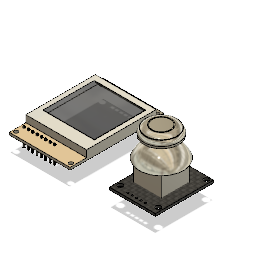
Paramotor_Instrument_Box-v4 (Autodesk Fusion 360 archive; units mm, degrees)
design "Burner Controller"
Autodesk Fusion 360 part; units mm, degrees
sketch "LCD_PCB" plane through (0, 0, 0) normal (0, 1, 0) x (1, 0, 0) in component "LCD Screen"
  line L0 (17.5, 27) -> (-17.5, 27)
  line L1 (-17.5, 27) -> (-17.5, -27)
  line L2 (-17.5, -27) -> (17.5, -27)
  line L3 (17.5, -27) -> (17.5, 27)
  line L4 (17.5, 27) -> (-17.5, -27) construction
  line L5 (-17.5, 27) -> (17.5, -27) construction
  circle A0 centre (-15.75, 24.75) radius 1.125
  circle A1 centre (15.75, 24.75) radius 1.125
  circle A2 centre (-15.75, -24.75) radius 1.125
  circle A3 centre (15.75, -24.75) radius 1.125
  circle A4 centre (0, 25) radius 0.5
  circle A5 centre (-10, 25) radius 0.5
  circle A6 centre (-7.5, 25) radius 0.5
  circle A7 centre (-5, 25) radius 0.5
  circle A8 centre (-2.5, 25) radius 0.5
  circle A9 centre (2.5, 25) radius 0.5
  circle A10 centre (5, 25) radius 0.5
  circle A11 centre (7.5, 25) radius 0.5
  circle A12 centre (10, 25) radius 0.5
  circle A13 centre (-15.5, -20) radius 0.5
  circle A14 centre (-13, -20) radius 0.5
  circle A15 centre (-10.5, -20) radius 0.5
  circle A16 centre (-8, -20) radius 0.5
  circle A17 centre (-5.5, -20) radius 0.5
  circle A18 centre (-3, -20) radius 0.5
  circle A19 centre (-0.5, -20) radius 0.5
  circle A20 centre (2, -20) radius 0.5
  dimension "d14" = 54
  dimension "d15" = 35
  dimension "d16" = 2.25
  dimension "d17" = 2.25
  dimension "d18" = 1.75
  dimension "d19" = 2.25
  dimension "d20" = 2.25
  dimension "d21" = 1.75
  dimension "d22" = 2.25
  dimension "d23" = 2.25
  dimension "d24" = 1.75
  dimension "d25" = 2.25
  dimension "d26" = 1.75
  dimension "d27" = 2.25
  dimension "d53" = 1
  dimension "d54" = 2
  dimension "d57" = 2.5
  dimension "d58" = 0
  dimension "d61" = 1
  dimension "d62" = 2
  dimension "d63" = 7
  dimension "d66" = 2.5
  dimension "d67" = 0
  constraint perpendicular L0 L1
  constraint parallel L0 L2
  constraint parallel L1 L3
  constraint horizontal L0
  constraint coincident L4 origin
  constraint coincident L5 origin
  measures "d14" distance of L0.end L1.end
  measures "d15" distance of L1.end L2.end
  measures "d16" diameter of A0
  measures "d17" distance of L0 A0.centre
  measures "d18" distance of L1 A0.centre
  measures "d19" diameter of A1
  measures "d20" distance of L0 A1.centre
  measures "d21" distance of L3 A1.centre
  measures "d22" diameter of A2
  measures "d23" distance of L2 A2.centre
  measures "d24" distance of L1 A2.centre
  measures "d25" diameter of A3
  measures "d26" distance of L3 A3.centre
  measures "d27" distance of L2 A3.centre
  measures "d53" diameter of A4
  measures "d54" distance of L0 A4.centre
  measures "d61" diameter of A13
  measures "d62" distance of L1 A13.centre
  measures "d63" distance of L2 A13.centre
extrude "Extrude1" add sketch "LCD_PCB" along normal blind 1.5 makes body 1 in component "LCD Screen"
sketch "LCD_Display" plane through (0, 1.5, 0) normal (0, 1, 0) x (-1, 0, 0) in component "LCD Screen"
  circle A0 centre (15.75, 24.75) radius 1.125
  circle A1 centre (-15.75, 24.75) radius 1.125
  circle A2 centre (-15.75, -24.75) radius 1.125
  circle A3 centre (15.75, -24.75) radius 1.125
  line L0 (-17.5, 27) -> (-17.5, -27)
  line L1 (-17.5, -27) -> (17.5, -27)
  line L2 (17.5, -27) -> (17.5, 27)
  line L3 (17.5, 27) -> (-17.5, 27)
  line L4 (-17.5, -22.5) -> (17.5, -22.5)
  line L5 (17.5, -22.5) -> (17.5, 17.5)
  line L6 (17.5, 17.5) -> (-17.5, 17.5)
  line L7 (-17.5, 17.5) -> (-17.5, -22.5)
  line L8 (-17.5, -22.5) -> (17.5, 17.5) construction
  line L9 (17.5, -22.5) -> (-17.5, 17.5) construction
  line L10 (14.75, -19.2) -> (-14.75, -19.2)
  line L11 (-14.75, -19.2) -> (-14.75, 10.3)
  line L12 (-14.75, 10.3) -> (14.75, 10.3)
  line L13 (14.75, 10.3) -> (14.75, -19.2)
  line L14 (14.75, -19.2) -> (-14.75, 10.3) construction
  line L15 (-14.75, -19.2) -> (14.75, 10.3) construction
  circle A4 centre (0, -25) radius 0.5
  circle A5 centre (-10, -25) radius 0.5
  circle A6 centre (-7.5, -25) radius 0.5
  circle A7 centre (-5, -25) radius 0.5
  circle A8 centre (-2.5, -25) radius 0.5
  circle A9 centre (2.5, -25) radius 0.5
  circle A10 centre (5, -25) radius 0.5
  circle A11 centre (7.5, -25) radius 0.5
  circle A12 centre (10, -25) radius 0.5
  circle A13 centre (-7.5, -25) radius 0.5
  circle A14 centre (-5, -25) radius 0.5
  circle A15 centre (-2.5, -25) radius 0.5
  circle A16 centre (-10, -25) radius 0.5
  circle A17 centre (2.5, -25) radius 0.5
  circle A18 centre (5, -25) radius 0.5
  circle A19 centre (7.5, -25) radius 0.5
  circle A20 centre (0, -25) radius 0.5
  circle A21 centre (10, -25) radius 0.5
  circle A22 centre (0.5, 20) radius 0.5
  circle A23 centre (-2, 20) radius 0.5
  circle A24 centre (13, 20) radius 0.5
  circle A25 centre (8, 20) radius 0.5
  circle A26 centre (5.5, 20) radius 0.5
  circle A27 centre (3, 20) radius 0.5
  circle A28 centre (10.5, 20) radius 0.5
  circle A29 centre (15.5, 20) radius 0.5
  point P0 (0, -2.5)
  point P1 (0, -4.45)
  dimension "d30" = 35
  dimension "d31" = 40
  dimension "d32" = 4.5
  dimension "d33" = 29.5
  dimension "d34" = 29.5
  dimension "d36" = 3.3
  dimension "d47" = 1
  dimension "d48" = 2
  dimension "d51" = 2.5
  dimension "d52" = 2.5
  constraint perpendicular L4 L5
  constraint parallel L4 L6
  constraint parallel L5 L7
  constraint horizontal L4
  constraint coincident L8 P0
  constraint coincident L9 P0
  constraint perpendicular L10 L11
  constraint parallel L10 L12
  constraint parallel L11 L13
  constraint horizontal L10
  constraint coincident L14 P1
  constraint coincident L15 P1
  measures "d30" distance of L5.end L6.end
  measures "d31" distance of L4.end L5.end
  measures "d32" distance of L1 L4
  measures "d33" distance of L11.end L12.end
  measures "d34" distance of L10.end L11.end
  measures "d36" distance of L4 L10
  measures "d47" diameter of A4
  measures "d48" distance of L1 A4.centre
extrude "Extrude2" add sketch "LCD_Display" along normal blind 4 contours L0 L2 L4 L5 L6 L7 bodies 1 in component "LCD Screen"
extrude "Extrude3" add 1 faces at (-4.9167, 1.5, -9.3667) along direction (0, 1, 0) blind 4.1 on bodies 1 bodies 1 in component "LCD Screen"
fillet "Fillet1" radius 0.1 4 edges at (0, 5.5, 10.3) (14.75, 5.5, -4.45) (0, 5.5, -19.2) (-14.75, 5.5, -4.45) on bodies 1 in component "LCD Screen"
sketch "Pins" plane through (0, 0, 0) normal (0, 1, 0) x (-1, 0, 0) in component "LCD Screen"
  line L0 (-16.5, 11.5) -> (-16.5, -21.5)
  line L1 (-16.5, -21.5) -> (16.5, -21.5)
  line L2 (16.5, -21.5) -> (16.5, 11.5)
  line L3 (16.5, 11.5) -> (-16.5, 11.5)
  line L4 (15.925, 20.075) -> (15.075, 20.075)
  line L5 (15.075, 20.075) -> (15.075, 20.925)
  line L6 (15.075, 20.925) -> (15.925, 20.925)
  line L7 (15.925, 20.925) -> (15.925, 20.075)
  line L8 (15.925, 20.075) -> (15.075, 20.925) construction
  line L9 (15.075, 20.075) -> (15.925, 20.925) construction
  line L10 (17.5, 17.5) -> (17.5, 27.5)
  line L11 (17.5, 27.5) -> (-17.5, 27.5)
  line L12 (13.425, 20.075) -> (12.575, 20.075)
  line L13 (13.425, 20.925) -> (13.425, 20.075)
  line L14 (12.575, 20.925) -> (13.425, 20.925)
  line L15 (12.575, 20.075) -> (12.575, 20.925)
  line L16 (10.925, 20.075) -> (10.075, 20.075)
  line L17 (10.925, 20.925) -> (10.925, 20.075)
  line L18 (10.075, 20.925) -> (10.925, 20.925)
  line L19 (10.075, 20.075) -> (10.075, 20.925)
  line L20 (8.425, 20.075) -> (7.575, 20.075)
  line L21 (8.425, 20.925) -> (8.425, 20.075)
  line L22 (7.575, 20.925) -> (8.425, 20.925)
  line L23 (7.575, 20.075) -> (7.575, 20.925)
  line L24 (5.925, 20.075) -> (5.075, 20.075)
  line L25 (5.925, 20.925) -> (5.925, 20.075)
  line L26 (5.075, 20.925) -> (5.925, 20.925)
  line L27 (5.075, 20.075) -> (5.075, 20.925)
  line L28 (3.425, 20.075) -> (2.575, 20.075)
  line L29 (3.425, 20.925) -> (3.425, 20.075)
  line L30 (2.575, 20.925) -> (3.425, 20.925)
  line L31 (2.575, 20.075) -> (2.575, 20.925)
  line L32 (0.925, 20.075) -> (0.075, 20.075)
  line L33 (0.925, 20.925) -> (0.925, 20.075)
  line L34 (0.075, 20.925) -> (0.925, 20.925)
  line L35 (0.075, 20.075) -> (0.075, 20.925)
  line L36 (-1.575, 20.075) -> (-2.425, 20.075)
  line L37 (-1.575, 20.925) -> (-1.575, 20.075)
  line L38 (-2.425, 20.925) -> (-1.575, 20.925)
  line L39 (-2.425, 20.075) -> (-2.425, 20.925)
  point P0 (15.5, 20.5)
  dimension "d68" = 0.85
  dimension "d69" = 0.85
  dimension "d70" = 2
  dimension "d71" = 7
  dimension "d75" = 0
  constraint perpendicular L4 L5
  constraint parallel L4 L6
  constraint parallel L5 L7
  constraint horizontal L4
  constraint coincident L8 P0
  constraint coincident L9 P0
  measures "d68" distance of L4.end L5.end
  measures "d69" distance of L5.end L6.end
  measures "d70" distance of P0 L10
  measures "d71" distance of P0 L11
extrude "Extrude4" add sketch "Pins" along normal blind 2.5 and the other way blind 8.5 separate body contours L4 L5 L6 L7 makes body 2 in component "LCD Screen"
chamfer "Chamfer1" distance 0.175 angle 45 12 edges at (-15.075, -3, 20.075) (-15.5, 2.5, 20.925) (-15.075, -8.5, 20.5) (-15.925, -8.5, 20.5) (-15.925, -3, 20.925) (-15.5, -8.5, 20.075) (-15.925, 2.5, 20.5) (-15.075, 2.5, 20.5) (-15.925, -3, 20.075) (-15.5, 2.5, 20.075) (-15.5, -8.5, 20.925) (-15.075, -3, 20.925) on bodies 2 in component "LCD Screen"
pattern_linear "R-Pattern1" count 8 spacing 2.5 along (1, 0, 0) of bodies 2 makes body 3 at (-13.0833, -1.225, 20.925) makes body 4 at (-10.5833, -1.225, 20.925) makes body 5 at (-8.0833, -1.225, 20.925) makes body 6 at (-5.5833, -1.225, 20.925) makes body 7 at (-3.0833, -1.225, 20.925) makes body 8 at (-0.5833, -1.225, 20.925) makes body 9 at (1.9167, -1.225, 20.925) in component "LCD Screen"
sketch "Joystick PCB" plane through (0, 0, 0) normal (0, 1, 0) x (1, 0, 0) in component "Navigation_Joystick"
  line L0 (20.1458, 8.0566) -> (-6.3542, 8.0566)
  line L1 (-6.3542, 8.0566) -> (-6.3542, -25.5434)
  circle A0 centre (-4.0542, 6.0566) radius 1.425
  line L2 (-6.3542, 8.0566) -> (20.1458, -25.5434) construction
  circle A1 centre (17.8458, 6.0566) radius 1.425
  line L3 (-6.3542, -25.5434) -> (20.1458, -25.5434)
  circle A2 centre (-4.0542, -21.5434) radius 1.425
  line L4 (20.1458, -25.5434) -> (20.1458, 8.0566)
  circle A3 centre (17.8458, -21.5434) radius 1.425
  circle A4 centre (6.8958, -23.0434) radius 0.5
  circle A5 centre (1.8958, -23.0434) radius 0.5
  circle A6 centre (4.3958, -23.0434) radius 0.5
  circle A7 centre (9.3958, -23.0434) radius 0.5
  circle A8 centre (11.8958, -23.0434) radius 0.5
  dimension "d95" = 33.6
  dimension "d96" = 26.5
  dimension "d97" = 2.85
  dimension "d98" = 2
  dimension "d99" = 2.3
  dimension "d100" = 2.85
  dimension "d101" = 2
  dimension "d102" = 2.3
  dimension "d103" = 2.85
  dimension "d104" = 4
  dimension "d105" = 2.3
  dimension "d106" = 2.85
  dimension "d107" = 2.3
  dimension "d108" = 4
  dimension "d118" = 1
  dimension "d120" = 2.5
  dimension "d123" = 2.5
  dimension "d124" = 0
  dimension "d167" = 13.25
  constraint perpendicular L0 L1
  constraint parallel L0 L3
  constraint parallel L1 L4
  constraint horizontal L0
  constraint coincident origin L2
  measures "d95" distance of L0.end L1.end
  measures "d96" distance of L2.end L1.end
  measures "d97" diameter of A0
  measures "d98" distance of A0.centre L0
  measures "d99" distance of A0.centre L1
  measures "d100" diameter of A1
  measures "d101" distance of A1.centre L0
  measures "d102" distance of A1.centre L4
  measures "d103" diameter of A2
  measures "d104" distance of A2.centre L3
  measures "d105" distance of A2.centre L1
  measures "d106" diameter of A3
  measures "d107" distance of A3.centre L4
  measures "d108" distance of A3.centre L3
  measures "d118" diameter of A4
  measures "d120" distance of L3 A4.centre
  measures "d167" distance of L1 A4.centre
extrude "Extrude1'" add sketch "Joystick PCB" along normal blind 1.5 separate body makes body 10 in component "Navigation_Joystick"
sketch "Pot Block" plane through (0, 0, 0) normal (0, 1, 0) x (-1, 0, 0) in component "Navigation_Joystick"
  line L0 (-13.9458, 15.9434) -> (2.0542, 15.9434)
  line L1 (2.0542, 15.9434) -> (2.0542, -0.0566)
  line L2 (2.0542, -0.0566) -> (-13.9458, -0.0566)
  line L3 (-13.9458, -0.0566) -> (-13.9458, 15.9434)
  line L4 (-13.9458, 15.9434) -> (2.0542, -0.0566) construction
  line L5 (2.0542, 15.9434) -> (-13.9458, -0.0566) construction
  line L6 (-20.1458, -8.0566) -> (6.3542, -8.0566)
  line L7 (6.3542, -8.0566) -> (6.3542, 25.5434)
  point P0 (-5.9458, 7.9434)
  dimension "d136" = 16
  dimension "d137" = 16
  dimension "d138" = 8
  dimension "d139" = 4.3
  constraint perpendicular L0 L1
  constraint parallel L0 L2
  constraint parallel L1 L3
  constraint horizontal L0
  constraint coincident L4 P0
  constraint coincident L5 P0
  measures "d136" distance of L1.end L2.end
  measures "d137" distance of L0.end L1.end
  measures "d138" distance of L2 L6
  measures "d139" distance of L1 L7
extrude "Extrude2'" add sketch "Pot Block" along normal blind 13.5 separate body makes body 11 in component "Navigation_Joystick"
ref_plane "WorkPlane1" through (6.8958, 9, 8.7434) normal (0, 1, 0) x (1, 0, 0) in component "Navigation_Joystick"
sketch "Joystick Knob" plane through (0, 9, 0) normal (0, 1, 0) x (1, 0, 0) in component "Navigation_Joystick"
  circle A0 centre (5.9458, -7.9434) radius 5.15
  point P0 (5.9458, -7.9434)
  dimension "d146" = 10.3
  constraint coincident P0 A0.centre
  measures "d146" diameter of A0
extrude "Extrude3'" add sketch "Joystick Knob" along normal blind 21 separate body makes body 12 in component "Navigation_Joystick"
cylinder "CylinderPrimitive1" add diameter 20 height -5 placed x (1, 0, 0) y (0, 0, -1) z (0, 1, 0) at (-1, 30, 0) separate body makes body 13 in component "Navigation_Joystick"
chamfer "Chamfer1'" distance 2.5 angle 45 1 edges at (2.6162, 30, 9.3233) on bodies 13 in component "Navigation_Joystick"
fillet "Fillet1'" radius 3.3333 1 edges at (-4.6162, 27.5, -9.3233) on bodies 13 in component "Navigation_Joystick"
fillet "Fillet2" radius 4.5455 1 edges at (1.7121, 30, -6.9925) on bodies 13 in component "Navigation_Joystick"
ref_plane "WorkPlane2" through (6.8958, 13.5, 8.7434) normal (0, 1, 0) x (1, 0, 0) in component "Navigation_Joystick"
move_body "Move1" bodies 13 to x (1, 0, 0) y (0, 1, 0) z (0, 0, 1) at (6.9458, 0, 7.9434) in component "Navigation_Joystick"
sketch "Sketch8" plane through (6.8958, 9, 8.7434) normal (0, 1, 0) x (1, 0, 0) in component "Navigation_Joystick"
  point P0 (-1, 0)
sphere "SpherePrimitive4" add diameter 27 placed x (1, 0, 0) y (0, 0, -1) z (0, 1, 0) at (5.9458, 9, 7.9434) separate body makes body 14 in component "Navigation_Joystick"
sphere "SpherePrimitive5" cut diameter 25.65 placed x (1, 0, 0) y (0, 0, -1) z (0, 1, 0) at (5.9458, 9, 7.9434) bodies 14 in component "Navigation_Joystick"
cylinder "CylinderPrimitive3" cut diameter 55 height -28 placed x (1, 0, 0) y (0, 0, -1) z (0, 1, 0) at (5.9458, 13.5, 7.9434) bodies 14 in component "Navigation_Joystick"
component "Burner Controller" placed x (1, 0, 0) y (0, 1, 0) z (0, 0, 1) at (0, 0, 0)
component "LCD Screen" placed x (1, 0, 0) y (0, 1, 0) z (0, 0, 1) at (0, 0, 0) in component "Burner Controller"
component "Navigation_Joystick" placed x (1, 0, 0) y (0, 1, 0) z (0, 0, 1) at (45, 0, 0) in component "Burner Controller"
equation "LCD_PCB_Width = 35 mm"
equation "LCD_PCB_Height = 54 mm"
equation "LCD_PCB_Thickness = 1.5 mm" comment "Just the board - not including chips/solder etc"
equation "LCD_PCB_Hole_Dia = 2.25 mm"
equation "LCD_PCB_Hole_Offset_Down_from_Top = 2.25 mm"
equation "LCD_PCB_Hole_Offest_in_from_Side = 1.75 mm"
equation "LCD_Display_Width = 35 mm"
equation "LCD_Display_Height = 40 mm"
equation "LCD_Display_Thickness = 4 mm" comment "Including gap between PCB and bottom of display"
equation "LCD_Display_Offest_Down_from_Top = 4.5 mm"
equation "LCD_Display_Visible_Width = 29.5 mm"
equation "LCD_Display_Visible_Height = 29.5 mm"
equation "LCD_Display_Visible_Offset_Down_from_Top_of_Display = 3.3 mm"
equation "d14 = LCD_PCB_Height"
equation "d15 = LCD_PCB_Width"
equation "d16 = LCD_PCB_Hole_Dia"
equation "d17 = LCD_PCB_Hole_Offset_Down_from_Top"
equation "d18 = LCD_PCB_Hole_Offest_in_from_Side"
equation "d19 = LCD_PCB_Hole_Dia"
equation "d20 = LCD_PCB_Hole_Offset_Down_from_Top"
equation "d21 = LCD_PCB_Hole_Offest_in_from_Side"
equation "d22 = LCD_PCB_Hole_Dia"
equation "d23 = LCD_PCB_Hole_Offset_Down_from_Top"
equation "d24 = LCD_PCB_Hole_Offest_in_from_Side"
equation "d25 = LCD_PCB_Hole_Dia"
equation "d26 = LCD_PCB_Hole_Offest_in_from_Side"
equation "d27 = LCD_PCB_Hole_Offset_Down_from_Top"
equation "d28 = LCD_PCB_Thickness"
equation "d30 = LCD_Display_Width"
equation "d31 = LCD_Display_Height"
equation "d32 = LCD_Display_Offest_Down_from_Top"
equation "d33 = LCD_Display_Visible_Width"
equation "d34 = LCD_Display_Visible_Height"
equation "d36 = LCD_Display_Visible_Offset_Down_from_Top_of_Display"
equation "d38 = LCD_Display_Thickness"
equation "d40 = LCD_Display_Thickness + 0.1 mm"
equation "Solder_Hole_Dia = 1 mm"
equation "Solder_Pitch = ( 20 / 8 ) * 1 mm"
equation "Num_Solder_Holes_Top = 9 mm" comment "Cannot have user parms for repeats :-("
equation "Top_Solder_Holes_Offest_Down_from_Top = 2 mm"
equation "d47 = Solder_Hole_Dia"
equation "d48 = Top_Solder_Holes_Offest_Down_from_Top"
equation "d51 = Solder_Pitch"
equation "d52 = Solder_Pitch"
equation "d53 = Solder_Hole_Dia"
equation "d54 = Top_Solder_Holes_Offest_Down_from_Top"
equation "d57 = Solder_Pitch"
equation "B_Solder_Hole_In_From_Left = 2 mm"
equation "B_Solder_Hole_Up_From_Bottom = 7 mm"
equation "d61 = Solder_Hole_Dia"
equation "d62 = B_Solder_Hole_In_From_Left"
equation "d63 = B_Solder_Hole_Up_From_Bottom"
equation "d66 = Solder_Pitch"
equation "d68 = Solder_Hole_Dia * 0.85"
equation "d69 = Solder_Hole_Dia * 0.85"
equation "d70 = B_Solder_Hole_In_From_Left"
equation "d71 = B_Solder_Hole_Up_From_Bottom"
equation "d74 = -Solder_Pitch"
equation "Pin_Height_Total = 11 mm"
equation "Pin_Protrusion_Amount = 8.5 mm"
equation "d78 = Pin_Height_Total - Pin_Protrusion_Amount"
equation "d80 = Pin_Protrusion_Amount"
equation "d82 = Solder_Hole_Dia * 0.175"
equation "d85 = Solder_Pitch"
equation "d95 = Joy_PCB_Height"
equation "d96 = Joy_PCB_Width"
equation "d97 = Joy_Hole_Dia"
equation "d98 = Joy_Hole_down_from_top"
equation "d99 = Joy_Hole_in_from_side"
equation "d100 = Joy_Hole_Dia"
equation "d101 = Joy_Hole_down_from_top"
equation "d102 = Joy_Hole_in_from_side"
equation "d103 = Joy_Hole_Dia"
equation "d104 = Joy_Hole_up_from_bottom"
equation "d105 = Joy_Hole_in_from_side"
equation "d106 = Joy_Hole_Dia"
equation "d107 = Joy_Hole_in_from_side"
equation "d108 = Joy_Hole_up_from_bottom"
equation "Joy_Hole_Dia = 2.85 mm"
equation "Joy_Hole_in_from_side = 2.3 mm"
equation "Joy_Hole_down_from_top = 2 mm"
equation "Joy_Hole_up_from_bottom = 4 mm"
equation "d118 = Solder_Hole_Dia"
equation "Joy_Solder_Holes_up_from_bottom = 2.5 mm"
equation "d120 = Joy_Solder_Holes_up_from_bottom"
equation "d123 = Solder_Pitch"
equation "Joy_PCB_thickness = 1.5 mm"
equation "d126 = Joy_PCB_thickness"
equation "Joy_Base_XY = 16 mm" comment "The silver cube holding the potentiometers that the joystick connects to"
equation "Joystick_Base_Sphere_Dia = 27 mm"
equation "Joystick_Base_Cut = Joystick_Base_Sphere_Dia / 1.7"
equation "Joystick_Cyl_Dia = 10.3 mm"
equation "Joystick_Top_Dia = 20 mm"
equation "Joystick_Top_Thickness = 5 mm"
equation "Joy_Base_down_from_top = 8 mm"
equation "Joy_Base_in_from_Left = 4.3 mm"
equation "d136 = Joy_Base_XY"
equation "d137 = Joy_Base_XY"
equation "d138 = Joy_Base_down_from_top"
equation "d139 = Joy_Base_in_from_Left"
equation "Joy_Base_Height = 12 mm"
equation "d141 = Joy_PCB_thickness + Joy_Base_Height"
equation "Pot_Pivot_up_from_PCB = 7.5 mm"
equation "Joystick_Cyl_Height = 21 mm" comment "total height of the joystick knob"
equation "d145 = Pot_Pivot_up_from_PCB"
equation "d146 = Joystick_Cyl_Dia"
equation "d147 = Joystick_Cyl_Height"
equation "d149 = -Joystick_Top_Thickness"
equation "d151 = Joystick_Top_Thickness / 2"
equation "d152 = Joystick_Top_Thickness / 1.5"
equation "d153 = Joystick_Top_Thickness / 1.1"
equation "Joystick_Basetop_Down_From_Sticktop = 17 mm"
equation "d157 = Joystick_Base_Sphere_Dia / 6"
equation "Joy_PCB_Height = 33.6 mm"
equation "Joy_PCB_Width = 26.5 mm"
equation "d163 = Joystick_Base_Sphere_Dia"
equation "d164 = Joystick_Base_Sphere_Dia * 0.95"
equation "d165 = -Joystick_Base_Sphere_Dia - 1 mm"
equation "d167 = Joy_PCB_Width / 2"
named bodies: "LCD", "pin", "pin (1)", "pin (2)", "pin (3)", "pin (4)", "pin (5)", "pin (6)", "pin (7)", "Joystick PCB", "Pot Block", "Joystick shaft", "Joystick knob", "Joystick base"

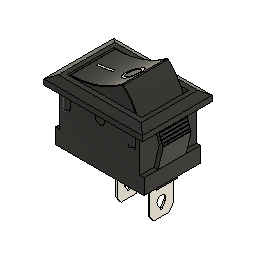
design "On Off Switch"
Autodesk Fusion 360 part; units mm, degrees
sketch "Sketch1" plane through (0, 0, 0) normal (0, 0, 1) x (1, 0, 0) in component "Body"
  line L0 (9.425, -6) -> (-9.425, -6)
  line L1 (-9.425, -6) -> (-9.425, 6)
  line L2 (-9.425, 6) -> (9.425, 6)
  line L3 (9.425, 6) -> (9.425, -6)
  line L4 (9.425, -6) -> (-9.425, 6) construction
  line L5 (-9.425, -6) -> (9.425, 6) construction
  line L6 (-8.55, 6) -> (8.55, 6)
  line L7 (8.55, 6) -> (8.55, -6)
  line L8 (8.55, -6) -> (-8.55, -6)
  line L9 (-8.55, -6) -> (-8.55, 6)
  line L10 (-8.55, 6) -> (8.55, -6) construction
  line L11 (8.55, 6) -> (-8.55, -6) construction
  dimension "d1" = 18.85
  dimension "d2" = 12
  dimension "d3" = 17.1
  dimension "d4" = 12
  constraint perpendicular L0 L1
  constraint parallel L0 L2
  constraint parallel L1 L3
  constraint horizontal L0
  constraint coincident L4 origin
  constraint coincident L5 origin
  constraint perpendicular L6 L7
  constraint parallel L6 L8
  constraint parallel L7 L9
  constraint horizontal L6
  constraint coincident L10 origin
  constraint coincident L11 origin
  measures "d1" distance of L1.end L2.end
  measures "d2" distance of L0.end L1.end
  measures "d3" distance of L7.end L8.end
  measures "d4" distance of L6.end L7.end
extrude "Extrude1" add sketch "Sketch1" along normal blind 3.3 contours L0 L2 L3 L7 | L0 L1 L2 L9 makes body 1 at (8.55, 2, 1.1) makes body 2 at (-8.55, -2, 1.1) in component "Body"
extrude "Extrude2" add sketch "Sketch1" along normal blind 11.2 contours L0 L2 L6 L7 L8 L9 bodies 1 2 in component "Body"
sketch "Sketch2" plane through (0, 6, 0) normal (0, 1, 0) x (-1, 0, 0) in component "Body"
  line L0 (-9.425, 0) -> (9.425, 0)
  line L1 (9.425, 0) -> (9.425, 3.3)
  line L2 (9.425, 3.3) -> (8.55, 3.3)
  line L3 (8.55, 3.3) -> (8.55, 11.2)
  line L4 (8.55, 11.2) -> (-8.55, 11.2)
  line L5 (-8.55, 11.2) -> (-8.55, 3.3)
  line L6 (-8.55, 3.3) -> (-9.425, 3.3)
  line L7 (-9.425, 3.3) -> (-9.425, 0)
  line L8 (-7.5905, 11.2) -> (-6.3405, 11.2)
  line L9 (-7.5905, 8.025) -> (-7.5905, 11.2)
  arc A0 (-7.5905, 8.025) -> (-6.9655, 7.4) centre (-6.9655, 8.025) ccw
  line L10 (-6.9655, 11.2) -> (-6.9655, 7.4)
  line L11 (0, 11.2) -> (0, 8.4604) construction
  line L12 (6.3405, 11.2) -> (6.3405, 8.025)
  arc A1 (6.3405, 8.025) -> (6.9655, 7.4) centre (6.9655, 8.025) ccw
  line L13 (6.9655, 11.2) -> (6.9655, 7.4)
  circle A2 centre (0, 9.35) radius 1
  line L14 (0, 9.35) -> (0, 0) construction
  dimension "d9" = 1.25
  dimension "d14" = 2
  dimension "d15" = 9.35
  constraint horizontal L8
  constraint vertical L9
  constraint coincident L4 L8.start
  constraint tangent L9 A0
  constraint midpoint L8 L10.start
  constraint midpoint L4 L11.start
  constraint perpendicular L4 L11
  constraint symmetric L8.end L11 L12.start
  constraint symmetric A0 L11 A1
  constraint symmetric L10.start L11 L13.start
  constraint symmetric A0.end L11 A1.end
  constraint coincident A2.centre L14.start
  constraint coincident L14.end origin
  constraint vertical L14
  measures "d9" distance of L8.start L8.end
  measures "d14" diameter of A2
  measures "d15" distance of A2.centre L14.end
revolve "Revolve1" add sketch "Sketch2" angle 360 about axis through (6.9655, 6, 11.2) along (0, 0, -1) contours L4 L8 L9 A0 L10 bodies 1 in component "Body"
revolve "Revolve2" add sketch "Sketch2" angle 360 about axis through (-6.9655, 6, 11.2) along (0, 0, -1) contours L4 L12 A1 L13 bodies 1 in component "Body"
mirror "Mirror1" about plane through (0, 0, 0) normal (0, 1, 0) of "Revolve1", "Revolve2" in component "Body"
extrude "Extrude5" cut sketch "Sketch2" against normal blind 12 contours A2 bodies 1 in component "Body"
sketch "Sketch3" plane through (0, 0, 0) normal (0, 0, -1) x (1, 0, 0) in component "Body"
  line L0 (-9.425, -6) -> (9.425, -6)
  line L1 (9.425, -6) -> (9.425, 6)
  line L2 (9.425, 6) -> (-9.425, 6)
  line L3 (-9.425, 6) -> (-9.425, -6)
  line L4 (-9.425, 2.225) -> (9.425, 2.225) construction
  line L5 (9.425, 2.225) -> (9.425, -2.225) construction
  line L6 (9.425, -2.225) -> (-9.425, -2.225) construction
  line L7 (-9.425, -2.225) -> (-9.425, 2.225) construction
  line L8 (-8.325, 2.225) -> (-7.275, 2.225)
  line L9 (-7.275, 2.225) -> (-7.275, -2.225)
  line L10 (-7.275, -2.225) -> (-8.325, -2.225)
  line L11 (-8.325, -2.225) -> (-8.325, 2.225)
  line L12 (-6.625, 2.225) -> (-5.575, 2.225)
  line L13 (-5.575, 2.225) -> (-5.575, -2.225)
  line L14 (-5.575, -2.225) -> (-6.625, -2.225)
  line L15 (-6.625, -2.225) -> (-6.625, 2.225)
  line L16 (-7.275, 0) -> (-6.625, 0) construction
  line L17 (-6.775, 3.275) -> (-7.125, 3.275)
  line L18 (-7.125, 3.275) -> (-7.125, -3.275)
  line L19 (-7.125, -3.275) -> (-6.775, -3.275)
  line L20 (-6.775, -3.275) -> (-6.775, 3.275)
  line L21 (-6.775, 3.275) -> (-7.125, -3.275) construction
  line L22 (-7.125, 3.275) -> (-6.775, -3.275) construction
  line L23 (8.325, 2.225) -> (8.325, -2.225) construction
  line L24 (-1.375, -2.225) -> (-1.375, 2.225)
  line L25 (-0.325, 2.225) -> (-0.325, -2.225)
  line L26 (-0.175, 3.275) -> (-0.175, -3.275)
  line L27 (0.175, -3.275) -> (0.175, 3.275)
  line L28 (0.325, -2.225) -> (0.325, 2.225)
  line L29 (1.375, 2.225) -> (1.375, -2.225)
  line L30 (-0.175, -3.275) -> (0.175, -3.275)
  line L31 (0.175, 3.275) -> (-0.175, 3.275)
  line L32 (5.575, -2.225) -> (5.575, 2.225)
  line L33 (6.625, 2.225) -> (6.625, -2.225)
  line L34 (6.775, 3.275) -> (6.775, -3.275)
  line L35 (7.125, -3.275) -> (7.125, 3.275)
  line L36 (7.275, -2.225) -> (7.275, 2.225)
  line L37 (8.325, 2.225) -> (8.325, -2.225)
  line L38 (6.775, -3.275) -> (7.125, -3.275)
  line L39 (7.125, 3.275) -> (6.775, 3.275)
  line L40 (-1.375, 2.225) -> (-0.325, 2.225)
  line L41 (-1.375, -2.225) -> (-0.325, -2.225)
  line L42 (0.325, -2.225) -> (1.375, -2.225)
  line L43 (0.325, 2.225) -> (1.375, 2.225)
  line L44 (5.575, 2.225) -> (6.625, 2.225)
  line L45 (5.575, -2.225) -> (6.625, -2.225)
  line L46 (7.275, -2.225) -> (8.325, -2.225)
  line L47 (7.275, 2.225) -> (8.325, 2.225)
  point P0 (-6.95, 0)
  dimension "d23" = 4.45
  dimension "d24" = 1.05
  dimension "d25" = 4.45
  dimension "d26" = 1.05
  dimension "d27" = 4.45
  dimension "d28" = 2.75
  dimension "d29" = 1.1
  dimension "d30" = 6.55
  dimension "d31" = 0.35
  dimension "d32" = 1.1
  dimension "d35" = 13.9
  dimension "d36" = 0
  constraint horizontal L4
  constraint vertical L5
  constraint horizontal L6
  constraint vertical L7
  constraint coincident L3 L4.start
  constraint midpoint L3 L7
  constraint horizontal L8
  constraint vertical L9
  constraint horizontal L10
  constraint vertical L11
  constraint coincident L4 L8.start
  constraint horizontal L12
  constraint vertical L13
  constraint horizontal L14
  constraint vertical L15
  constraint coincident L4 L12.start
  constraint midpoint L9 L16.start
  constraint midpoint L15 L16.end
  constraint perpendicular L17 L18
  constraint parallel L17 L19
  constraint parallel L18 L20
  constraint horizontal L17
  constraint coincident L21 P0
  constraint coincident L22 P0
  constraint midpoint L16 P0
  constraint coincident L4 L23.start
  constraint coincident L6 L23.end
  constraint perpendicular L6 L23
  measures "d23" distance of L4.start L6.end
  measures "d24" distance of L8.start L8.end
  measures "d25" distance of L8.start L10.end
  measures "d26" distance of L12.start L12.end
  measures "d27" distance of L12.start L14.end
  measures "d28" distance of L11 L13
  measures "d29" distance of L7 L11
  measures "d30" distance of L17.end L18.end
  measures "d31" distance of L18.end L19.end
  measures "d32" distance of L5 L23
extrude "Extrude6" add sketch "Sketch3" along normal blind 1.4 contours L8 L9 L10 L11 | L12 L13 L14 L15 | L24 L25 L40 L41 | L28 L29 L42 L43 | L32 L33 L44 L45 | L36 L37 L46 L47 bodies 1 in component "Body"
sketch "Sketch4" plane through (0, 0, 11.2) normal (0, 0, 1) x (-1, 0, 0) in component "Body"
  line L0 (6.3405, 6) -> (-6.3405, 6)
  arc A0 (-6.3405, 6) -> (-7.5905, 6) centre (-6.9655, 6) ccw
  line L1 (-7.5905, 6) -> (-8.55, 6)
  line L2 (-8.55, 6) -> (-8.55, -6)
  line L3 (-8.55, -6) -> (-7.5905, -6)
  arc A1 (-7.5905, -6) -> (-6.3405, -6) centre (-6.9655, -6) ccw
  line L4 (-6.3405, -6) -> (6.3405, -6)
  arc A2 (6.3405, -6) -> (7.5905, -6) centre (6.9655, -6) ccw
  line L5 (7.5905, -6) -> (8.55, -6)
  line L6 (8.55, -6) -> (8.55, 6)
  line L7 (8.55, 6) -> (7.5905, 6)
  arc A3 (7.5905, 6) -> (6.3405, 6) centre (6.9655, 6) ccw
  line L8 (-10.5, 7.45) -> (10.5, 7.45)
  line L9 (10.5, 7.45) -> (10.5, -7.45)
  line L10 (10.5, -7.45) -> (-10.5, -7.45)
  line L11 (-10.5, -7.45) -> (-10.5, 7.45)
  line L12 (-10.5, 7.45) -> (10.5, -7.45) construction
  line L13 (10.5, 7.45) -> (-10.5, -7.45) construction
  dimension "d41" = 21
  dimension "d42" = 14.9
  constraint perpendicular L8 L9
  constraint parallel L8 L10
  constraint parallel L9 L11
  constraint horizontal L8
  constraint coincident L12 origin
  constraint coincident L13 origin
  measures "d41" distance of L9.end L10.end
  measures "d42" distance of L8.end L9.end
extrude "Extrude8" add sketch "Sketch4" along normal blind 1.15 contours L0 A0 L1 L2 L3 A1 L4 A2 L5 L6 L7 A3 | L8 L9 L10 L11 bodies 1 in component "Body"
ref_plane "WorkPlane1" through (0, 0, 13.2) normal (0, 0, 1) x (1, 0, 0) in component "Body"
sketch "Sketch5" plane through (0, 0, 13.2) normal (0, 0, 1) x (1, 0, 0) in component "Body"
  line L0 (8.85, -6) -> (-8.85, -6)
  line L1 (-8.85, -6) -> (-8.85, 6)
  line L2 (-8.85, 6) -> (8.85, 6)
  line L3 (8.85, 6) -> (8.85, -6)
  line L4 (8.85, -6) -> (-8.85, 6) construction
  line L5 (-8.85, -6) -> (8.85, 6) construction
  line L6 (-7.95, -5) -> (7.95, -5)
  line L7 (7.95, -5) -> (7.95, 5)
  line L8 (7.95, 5) -> (-7.95, 5)
  line L9 (-7.95, 5) -> (-7.95, -5)
  line L10 (-7.95, -5) -> (7.95, 5) construction
  line L11 (7.95, -5) -> (-7.95, 5) construction
  dimension "d46" = 17.7
  dimension "d47" = 12
  dimension "d48" = 15.9
  dimension "d49" = 10
  constraint perpendicular L0 L1
  constraint parallel L0 L2
  constraint parallel L1 L3
  constraint horizontal L0
  constraint coincident L4 origin
  constraint coincident L5 origin
  constraint perpendicular L6 L7
  constraint parallel L6 L8
  constraint parallel L7 L9
  constraint horizontal L6
  constraint coincident L10 origin
  constraint coincident L11 origin
  measures "d46" distance of L1.end L2.end
  measures "d47" distance of L0.end L1.end
  measures "d48" distance of L7.end L8.end
  measures "d49" distance of L6.end L7.end
loft "Loft1" add profiles "Sketch5" section 1 face at (3.5, -2.4833, 12.35) section 2 on bodies 1 bodies 1 in component "Body"
extrude "Extrude9" cut sketch "Sketch5" against normal blind 12.125 contours L6 L7 L8 L9 bodies 1 in component "Body"
extrude "Extrude10" cut sketch "Sketch3" against normal blind 1.075 contours L17 L18 L19 L20 | L26 L27 L30 L31 | L34 L35 L38 L39 bodies 1 in component "Body"
sketch "Sketch6" plane through (0, 0, 0) normal (0, 1, 0) x (1, 0, 0) in component "Body"
  circle A0 centre (0, -9.35) radius 1 construction
  line L0 (-6.3405, -11.2) -> (-6.3405, -8.025) construction
  arc A1 (-6.3405, -8.025) -> (-7.5905, -8.025) centre (-6.9655, -8.025) ccw construction
  line L1 (-7.5905, -8.025) -> (-7.5905, -11.2) construction
  line L2 (-7.5905, -11.2) -> (-8.55, -11.2) construction
  line L3 (-8.55, -11.2) -> (-8.55, -3.3) construction
  line L4 (-8.55, -3.3) -> (-9.425, -3.3) construction
  line L5 (-9.425, -3.3) -> (-9.425, 0) construction
  line L6 (-9.425, 0) -> (9.425, 0) construction
  line L7 (9.425, 0) -> (9.425, -3.3) construction
  line L8 (9.425, -3.3) -> (8.55, -3.3)
  line L9 (8.55, -3.3) -> (8.55, -11.2) construction
  line L10 (8.55, -11.2) -> (7.5905, -11.2) construction
  line L11 (7.5905, -11.2) -> (7.5905, -8.025) construction
  arc A2 (7.5905, -8.025) -> (6.3405, -8.025) centre (6.9655, -8.025) ccw construction
  line L12 (6.3405, -8.025) -> (6.3405, -11.2) construction
  line L13 (6.3405, -11.2) -> (-6.3405, -11.2) construction
  line L14 (-10.5, -11.2) -> (10.5, -11.2) construction
  line L15 (10.5, -11.2) -> (10.5, -12.35) construction
  line L16 (10.5, -12.35) -> (-10.5, -12.35) construction
  line L17 (-10.5, -12.35) -> (-10.5, -11.2) construction
  line L18 (10.5, -11.2) -> (10.5, 0.0232) construction
  line L19 (9.425, -3.3) -> (10.5, -8)
  line L20 (8.55, -3.3) -> (9.625, -8)
  line L21 (9.625, -8) -> (8.55, -11.2)
  line L22 (10.5, -8) -> (9.425, -11.2) construction
  line L23 (10.3609, -8) -> (10.5, -8)
  line L24 (10.3609, -8) -> (10.3609, -8.414)
  line L25 (10.3609, -8.414) -> (10.1609, -8.4146)
  line L26 (10.1609, -8.4146) -> (10.1625, -9.0047)
  line L27 (10.1625, -9.0047) -> (9.9625, -9.0052)
  line L28 (9.9625, -9.0052) -> (9.9625, -9.6)
  line L29 (9.9625, -9.6) -> (9.7625, -9.6)
  line L30 (9.7625, -9.6) -> (9.7625, -10.1953)
  line L31 (9.7625, -10.1953) -> (9.5625, -10.1953)
  line L32 (9.5625, -10.1953) -> (9.5625, -10.7907)
  line L33 (9.5625, -10.7907) -> (9.3625, -10.7907)
  line L34 (9.3625, -10.7907) -> (9.3625, -11.2)
  line L35 (8.55, -11.2) -> (9.3625, -11.2)
  dimension "d54" = 4.7
  dimension "d55" = 0.2
  dimension "d56" = 0.2
  dimension "d57" = 0.2
  dimension "d58" = 0.2
  dimension "d59" = 0.2
  constraint coincident L14.end L15.start
  constraint perpendicular L14 L18
  constraint coincident L7.end L8.start
  constraint coincident L18 L19.end
  constraint coincident L8.end L9.start
  constraint parallel L19 L20
  constraint coincident L9.end L10.start
  constraint coincident L14 L22.end
  constraint parallel L21 L22
  constraint perpendicular L18 L23
  constraint coincident L22 L24.end
  constraint perpendicular L23 L24
  constraint coincident L22 L26.end
  constraint perpendicular L25 L26
  constraint perpendicular L26 L27
  constraint midpoint L22 L28.end
  constraint coincident L22 L30.end
  constraint perpendicular L29 L30
  constraint coincident L22 L32.end
  constraint perpendicular L31 L32
  constraint coincident L14 L34.end
  constraint perpendicular L14 L34
  constraint vertical L28
  measures "d54" vertical distance of L7.end L19.end
  measures "d55" distance of L24.end L25.end
  measures "d56" distance of L26.end L27.end
  measures "d57" distance of L28.end L29.end
  measures "d58" distance of L30.end L31.end
  measures "d59" distance of L32.end L33.end
extrude "Extrude11" add sketch "Sketch6" along normal mid plane 6 bodies 1 in component "Body"
mirror "Mirror2" about plane through (0, 0, 0) normal (1, 0, 0) of "Extrude11" in component "Body"
sketch "Sketch1 (2)" plane through (0, 0, 0) normal (0, 1, 0) x (1, 0, 0) in component "Switch"
  circle A0 centre (0, -9.35) radius 1
  line L0 (8.85, -13.2) -> (-8.85, -13.2)
  line L1 (-8.55, -3.3) -> (-8.55, -11.2)
  line L2 (8.55, -3.3) -> (8.55, -11.2)
  arc A1 (-7.5504, -9.754) -> (-6.0755, -15.3373) centre (5.2198, -9.3671) ccw
  line L3 (0, -9.35) -> (0, -13.2) construction
  arc A2 (6.0755, -15.3373) -> (7.5504, -9.754) centre (-5.2198, -9.3671) ccw
  arc A3 (5.7771, -15.4582) -> (-5.7771, -15.4582) centre (0, -33.208) ccw
  arc A4 (-6.0755, -15.3373) -> (-5.7771, -15.4582) centre (-5.8545, -15.2205) ccw
  arc A5 (5.7771, -15.4582) -> (6.0755, -15.3373) centre (5.8545, -15.2205) ccw
  circle A6 centre (0, -9.35) radius 0.95
  arc A7 (7.5504, -9.754) -> (-7.5504, -9.754) centre (0, -9.5252) ccw
  dimension "d63" = 0.25
  dimension "d68" = 1.9
  constraint coincident A0.centre L3.start
  constraint midpoint L0 L3.end
  constraint symmetric A1.start L3 A2.end
  constraint symmetric A1 L3 A2
  constraint tangent A2 A5
  constraint tangent A3 A5
  constraint equal A4 A5
  constraint tangent A1 A7
  measures "d63" radius of A4
  measures "d68" diameter of A6
extrude "Extrude1'" add sketch "Sketch1 (2)" along normal mid plane 9.7 separate body contours L0 A1 A2 A3 A4 A5 | L0 A1 A2 A7 makes body 3 in component "Switch"
extrude "Extrude3" add sketch "Sketch1 (2)" along normal mid plane 12 separate body contours A6 makes body 4 in component "Switch"
extrude "Extrude4" add sketch "Sketch1 (2)" along normal mid plane 9.7 contours A0 bodies 3 4 in component "Switch"
sketch "Sketch1 (3)" plane through (7.125, 0, 0) normal (-1, 0, 0) x (0, -1, 0) in component "Pins"
  line L0 (-3.275, 0) -> (3.275, 0)
  line L1 (3.275, 0) -> (3.275, 1.075)
  line L2 (3.275, 1.075) -> (-3.275, 1.075)
  line L3 (-3.275, 1.075) -> (-3.275, 0)
  line L4 (2.225, 0) -> (2.225, -1.4)
  line L5 (-2.225, 0) -> (-2.225, -1.4)
  line L6 (2.225, -1.4) -> (-2.225, -1.4)
  line L7 (6, 0) -> (-6, 0)
  line L8 (-3.275, 0) -> (-3.275, 1.075)
  line L9 (3.275, 0) -> (3.275, 1.075)
  line L10 (-2.475, 0) -> (2.475, 0)
  line L11 (2.475, 0) -> (2.475, -8)
  line L12 (2.475, -8) -> (-2.475, -8)
  line L13 (-2.475, -8) -> (-2.475, 0)
  arc A0 (-2.475, 0) -> (-2.927, 0.2143) centre (-2.7518, 0) ccw
  line L14 (-2.927, 0.2143) -> (-3.4667, -0.2272)
  arc A1 (-3.8869, 0) -> (-3.4667, -0.2272) centre (-3.6302, -0.0273) ccw
  line L15 (-3.8869, 0) -> (-3.8869, 0.5375)
  line L16 (-3.8869, 0.5375) -> (0, 0.5375)
  line L17 (0, 0.5375) -> (0, 0) construction
  arc A2 (2.927, 0.2143) -> (2.475, 0) centre (2.7518, 0) ccw
  line L18 (2.927, 0.2143) -> (3.4667, -0.2272)
  arc A3 (3.4667, -0.2272) -> (3.8869, 0) centre (3.6302, -0.0273) ccw
  line L19 (3.8869, 0) -> (3.8869, 0.5375)
  line L20 (3.8869, 0.5375) -> (0, 0.5375)
  line L21 (1.6286, -8) -> (2.475, -6.781)
  line L22 (-1.6286, -8) -> (-2.475, -6.781)
  line L23 (0, -8) -> (0, 0) construction
  line L24 (-0.8182, -5.4791) -> (-0.2056, -6.5177)
  line L25 (0.8182, -5.4791) -> (0.2056, -6.5177)
  arc A4 (-0.2056, -6.5177) -> (0.2056, -6.5177) centre (0, -6.3964) ccw
  arc A5 (0.8182, -5.4791) -> (-0.8182, -5.4791) centre (0, -4.9964) ccw
  dimension "d80" = 4.95
  dimension "d81" = 8
  dimension "d82" = 6.6
  dimension "d83" = 1.9
  dimension "d84" = 1.4
  constraint horizontal L10
  constraint vertical L11
  constraint horizontal L12
  constraint vertical L13
  constraint midpoint L0 L10
  constraint tangent L13 A0
  constraint tangent A0 L14
  constraint coincident L7 A1.start
  constraint tangent L14 A1
  constraint perpendicular L7 L15
  constraint perpendicular L15 L16
  constraint coincident L17.end L23.end
  constraint perpendicular L10 L17
  constraint symmetric L10.start L17 L10.end
  constraint symmetric A0.end L17 A2.start
  constraint symmetric A0 L17 A2
  constraint symmetric L14.end L17 L18.end
  constraint symmetric A1.start L17 A3.end
  constraint symmetric A1 L17 A3
  constraint symmetric L15.end L17 L19.end
  constraint symmetric L16.end L17 L20.end
  constraint coincident L12 L21.start
  constraint symmetric L17 L21.start L22.start
  constraint symmetric L17 L21.end L22.end
  constraint midpoint L12 L23.start
  constraint coincident A5.centre L23
  constraint tangent L24 A5
  constraint symmetric L23 L24.start L25.start
  constraint tangent L24 A4
  constraint tangent L25 A4
  constraint coincident L23 A4.centre
  measures "d80" distance of L10.start L10.end
  measures "d81" distance of L10.start L12.end
  measures "d82" distance of L6 L12
  measures "d83" diameter of A5
  measures "d84" distance of A5.centre A4.centre
extrude "Extrude1''" add sketch "Sketch1 (3)" along normal blind 0.35 separate body contours L0 L1 L3 L7 L8 L9 L10 A0 L14 L16 A2 L18 L20 | L0 L4 L5 L6 L7 L10 L11 L12 L13 L21 L22 | L0 L4 L5 L6 L7 L10 | L0 L7 L14 A1 | L3 L7 L8 L15 L16 | L0 L7 L18 A3 | L1 L7 L9 L19 L20 makes body 5 in component "Pins"
extrude "Extrude2'" add sketch "Sketch1 (3)" along normal blind 0.35 from surface at 6.95 separate body contours L0 L1 L3 L7 L8 L9 L10 A0 L14 L16 A2 L18 L20 | L0 L4 L5 L6 L7 L10 L11 L12 L13 L21 L22 | L0 L4 L5 L6 L7 L10 | L0 L7 L14 A1 | L3 L7 L8 L15 L16 | L0 L7 L18 A3 | L1 L7 L9 L19 L20 makes body 6 in component "Pins"
fillet "Fillet1" radius 0.1 12 edges at (-7.1326, -4.85, 12.6301) (0, -4.85, 1.9714) (7.1326, -4.85, 12.6301) (5.9484, -4.85, 15.4522) (0, -4.85, 14.5417) (-5.9484, -4.85, 15.4522) (7.1326, 4.85, 12.6301) (0, 4.85, 1.9714) (-7.1326, 4.85, 12.6301) (-5.9484, 4.85, 15.4522) (0, 4.85, 14.5417) (5.9484, 4.85, 15.4522) on bodies 3 in component "Switch"
ref_plane "WorkPlane1" through (5.7771, 4.75, 15.4582) normal (0, 0, 1) x (1, 0, 0) in component "Switch"
sketch "Sketch2 (2)" plane through (5.7771, 4.75, 15.4582) normal (0, 0, 1) x (1, 0, 0) in component "Switch"
  line L0 (-11.5542, 0) -> (0, 0)
  line L1 (-11.5542, 0) -> (-11.5542, -9.5)
  line L2 (0, -9.5) -> (-11.5542, -9.5)
  line L3 (0, -9.5) -> (0, 0)
  line L4 (0, -4.75) -> (-11.5542, -4.75) construction
  line L5 (-5.7771, 0) -> (-5.7771, -9.5) construction
  circle A0 centre (-2.6872, -4.75) radius 1.8996
  circle A1 centre (-2.6872, -4.75) radius 1.3996
  line L6 (-10.6166, -4.5) -> (-7.1166, -4.5)
  line L7 (-7.1166, -4.5) -> (-7.1166, -5)
  line L8 (-7.1166, -5) -> (-10.6166, -5)
  line L9 (-10.6166, -5) -> (-10.6166, -4.5)
  line L10 (-10.6166, -4.5) -> (-7.1166, -5) construction
  line L11 (-7.1166, -4.5) -> (-10.6166, -5) construction
  point P0 (-8.8666, -4.75)
  dimension "d91" = 0.5
  dimension "d92" = 3.5
  dimension "d93" = 0.5
  constraint midpoint L3 L4.start
  constraint midpoint L1 L4.end
  constraint midpoint L0 L5.start
  constraint midpoint L2 L5.end
  constraint coincident L4 A0.centre
  constraint perpendicular L6 L7
  constraint parallel L6 L8
  constraint parallel L7 L9
  constraint horizontal L6
  constraint coincident L10 P0
  constraint coincident L11 P0
  constraint coincident L4 P0
  measures "d92" distance of L7.end L8.end
  measures "d93" distance of L6.end L7.end
extrude "Extrude5'" add sketch "Sketch2 (2)" along normal blind 0.01 from the near side of the face at (5.0276, -1.5833, 15.2315) contours A0 on bodies 3 bodies 3 in component "Switch"
extrude "Extrude6'" add sketch "Sketch2 (2)" along normal blind 0.01 from the near side of the face at (-0.386, -0.0111, 14.5457) contours L6 L7 L8 L9 on bodies 3 bodies 3 in component "Switch"
component "Body" placed x (1, 0, 0) y (0, 1, 0) z (0, 0, 1) at (0, 0, 0)
component "Switch" placed x (0.945519, 0, 0.325568) y (0, 1, 0) z (-0.325568, 0, 0.945519) at (3.0441, 0, 0.5094)
component "Pins" placed x (1, 0, 0) y (0, 1, 0) z (0, 0, 1) at (0, 0, 0)
